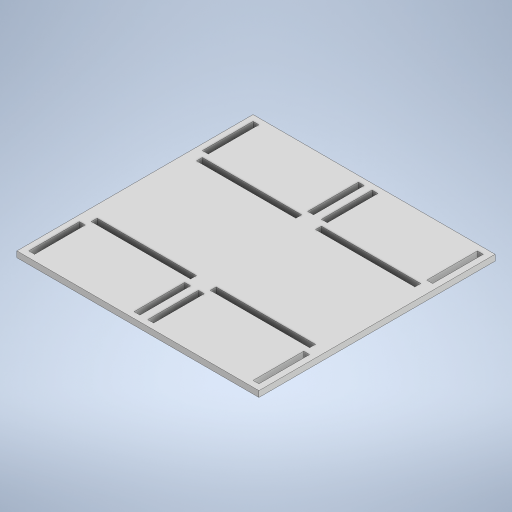
# Autodesk Inventor part: top
Saved by Autodesk Inventor 2023 (Build 270158000, 158)
## iProperties
Created: 2023-11-13
Part Number: top
Material: Generic
Document SubType Name: Modeling
Designer: Nate
Density: 1 g/cm^3
Appearance: Default
Mass: 45.5982 g
Surface Area: 339.233 cm^2
Volume: 45.5982 cm^3
Author: Nate
Autodesk Inventor part; units mm, degrees
ref_plane "YZ Plane" through (0, 0, 0) normal (1, 0, 0) x (0, 1, 0)
ref_plane "XZ Plane" through (0, 0, 0) normal (0, 1, 0) x (-1, 0, 0)
ref_plane "XY Plane" through (0, 0, 0) normal (0, 0, 1) x (1, 0, 0)
sketch "Sketch1" plane through (0, 0, 0) normal (0, 1, 0) x (-1, 0, 0)
  line L0 (0, 0) -> (127, 0)
  line L1 (127, 0) -> (127, -127)
  line L2 (127, -127) -> (0, -127)
  line L3 (0, -127) -> (0, 0)
  line L4 (123.825, 0) -> (127, 0)
  line L5 (127, 0) -> (127, -33.615)
  line L6 (127, -33.615) -> (123.825, -33.615)
  line L7 (123.825, -33.615) -> (123.825, 0)
  line L8 (123.825, -33.615) -> (70.363, -33.615)
  line L9 (70.363, -33.615) -> (70.363, -36.79)
  line L10 (70.363, -36.79) -> (127, -36.79)
  line L11 (70.363, -36.79) -> (67.188, -36.79)
  line L12 (67.188, -36.79) -> (67.188, 0)
  line L13 (67.188, 0) -> (70.363, 0)
  line L14 (70.363, 0) -> (70.363, -36.79)
  line L15 (127, -90.21) -> (67.188, -90.21)
  line L16 (67.188, -90.21) -> (67.188, -93.385)
  line L17 (67.188, -93.385) -> (127, -93.385)
  line L18 (127, -93.385) -> (127, -90.21)
  line L19 (127, -93.385) -> (123.825, -93.385)
  line L20 (123.825, -93.385) -> (123.825, -127)
  line L21 (123.825, -127) -> (127, -127)
  line L22 (127, -127) -> (127, -93.385)
  line L23 (25.4, 0) -> (6.35, 0)
  line L24 (25.4, -127) -> (6.35, -127)
  line L25 (67.188, -90.21) -> (70.363, -90.21)
  line L26 (70.363, -90.21) -> (70.363, -127)
  line L27 (70.363, -127) -> (67.188, -127)
  line L28 (67.188, -127) -> (67.188, -90.21)
  line L29 (67.188, -3.175) -> (70.363, -3.175)
  line L30 (70.363, -3.175) -> (70.363, -33.615)
  line L31 (70.363, -33.615) -> (67.188, -33.615)
  line L32 (67.188, -33.615) -> (67.188, -3.175)
  line L33 (73.538, -33.615) -> (123.825, -33.615)
  line L34 (123.825, -33.615) -> (123.825, -36.79)
  line L35 (123.825, -36.79) -> (73.538, -36.79)
  line L36 (127, -3.175) -> (123.825, -3.175)
  line L37 (123.825, -3.175) -> (123.825, -30.44)
  line L38 (123.825, -30.44) -> (127, -30.44)
  line L39 (127, -30.44) -> (127, -3.175)
  line L40 (123.825, -90.21) -> (81.7068, -90.21)
  line L41 (81.7068, -93.385) -> (123.825, -93.385)
  line L42 (123.825, -93.385) -> (123.825, -90.21)
  line L43 (123.825, -96.56) -> (127, -96.56)
  line L44 (127, -96.56) -> (127, -123.825)
  line L45 (127, -123.825) -> (123.825, -123.825)
  line L46 (123.825, -123.825) -> (123.825, -96.56)
  line L47 (70.363, -96.56) -> (67.188, -96.56)
  line L48 (67.188, -96.56) -> (67.188, -123.825)
  line L49 (67.188, -123.825) -> (70.363, -123.825)
  line L50 (70.363, -123.825) -> (70.363, -96.56)
  line L51 (70.363, -30.44) -> (67.188, -30.44)
  line L52 (22.225, 0) -> (9.525, 0)
  line L53 (9.525, -127) -> (22.225, -127)
  line L54 (127, 0) -> (130.175, 0)
  line L55 (130.175, 0) -> (130.175, -127)
  line L56 (130.175, -127) -> (127, -127)
  line L57 (127, -127) -> (127, 0)
  line L58 (3.175, 0) -> (0, 0)
  line L59 (0, 0) -> (0, -127)
  line L60 (0, -127) -> (3.175, -127)
  line L61 (3.175, -127) -> (3.175, 0)
  line L62 (62.987, 0) -> (62.987, -33.6042)
  line L63 (62.987, -33.6042) -> (59.812, -33.6042)
  line L64 (59.812, -33.6042) -> (59.812, -4.3263)
  line L65 (59.812, -33.6042) -> (6.35, -33.6042)
  line L66 (6.35, -33.6042) -> (6.35, -36.7792)
  line L67 (6.35, -36.7792) -> (62.987, -36.7792)
  line L68 (6.35, -36.7792) -> (3.175, -36.7792)
  line L69 (3.175, -36.7792) -> (3.175, -2.1822)
  line L70 (6.35, 0) -> (6.35, -36.7792)
  line L71 (3.175, -3.175) -> (6.35, -3.175)
  line L72 (6.35, -3.175) -> (6.35, -33.6042)
  line L73 (6.35, -33.6042) -> (3.175, -33.6042)
  line L74 (3.175, -33.6042) -> (3.175, -3.175)
  line L75 (59.812, -33.6042) -> (59.812, -36.7792)
  line L76 (62.987, -3.175) -> (59.812, -3.175)
  line L77 (59.812, -3.175) -> (59.812, -30.4292)
  line L78 (59.812, -30.4292) -> (62.987, -30.4292)
  line L79 (62.987, -30.4292) -> (62.987, -3.175)
  line L80 (6.35, -30.4292) -> (3.175, -30.4292)
  line L81 (62.987, -36.7792) -> (62.987, 0)
  line L82 (59.812, -3.175) -> (59.812, 0)
  line L83 (62.992, -127) -> (59.817, -127)
  line L84 (59.817, -127) -> (59.817, -90.2208)
  line L85 (59.817, -90.2208) -> (62.992, -90.2208)
  line L86 (62.992, -90.2208) -> (62.992, -127)
  line L87 (62.992, -93.3958) -> (3.175, -93.3958)
  line L88 (3.175, -93.3958) -> (3.175, -90.2208)
  line L89 (3.175, -90.2208) -> (62.992, -90.2208)
  line L90 (62.992, -90.2208) -> (62.992, -93.3958)
  line L91 (6.35, -90.2208) -> (3.175, -90.2208)
  line L92 (3.175, -90.2208) -> (3.175, -127)
  line L93 (3.175, -127) -> (6.35, -127)
  line L94 (6.35, -127) -> (6.35, -90.2208)
  line L95 (6.35, -123.825) -> (3.175, -123.825)
  line L96 (3.175, -123.825) -> (3.175, -96.5708)
  line L97 (3.175, -96.5708) -> (6.35, -96.5708)
  line L98 (6.35, -96.5708) -> (6.35, -123.825)
  line L99 (62.992, -123.825) -> (59.817, -123.825)
  line L100 (59.817, -123.825) -> (59.817, -96.5708)
  line L101 (59.817, -96.5708) -> (62.992, -96.5708)
  line L102 (62.992, -96.5708) -> (62.992, -123.825)
  point P0 (97.094, -33.615)
  point P1 (123.825, -110.1925)
  point P2 (123.825, -16.8075)
  point P3 (125.4125, 0)
  point P4 (125.4125, -3.175)
  point P5 (125.4125, -33.615)
  point P6 (70.363, -35.2025)
  point P7 (68.7755, -36.79)
  point P8 (68.7755, -33.615)
  point P9 (68.7755, 0)
  point P10 (68.7755, -3.175)
  point P11 (68.7755, -127)
  point P12 (68.7755, -123.825)
  point P13 (70.363, -93.385)
  point P14 (70.363, -30.44)
  point P15 (127, -96.56)
  point P16 (127, -30.44)
  point P17 (123.825, -33.615)
  point P18 (67.188, -96.56)
  point P19 (127, -93.385)
  point P20 (33.081, -33.6042)
  point P21 (59.812, -18.9652)
  point P22 (61.3995, -3.175)
  point P23 (61.3995, -33.6042)
  point P24 (6.35, -35.1917)
  point P25 (4.7625, -36.7792)
  point P26 (4.7625, -33.6042)
  point P27 (4.7625, -3.175)
  point P28 (59.817, -93.3958)
  point P29 (6.35, -93.3958)
  point P30 (3.175, -3.175)
  dimension "d0" = 127
  dimension "d2" = 127
  dimension "d5" = 33.615
  dimension "d6" = 33.615
  dimension "d7" = 53.462
  dimension "d8" = 53.462
  dimension "d9" = 3.175
  dimension "d10" = 3.175
  dimension "d11" = 3.175
  dimension "d12" = 3.175
  dimension "d13" = 3.175
  dimension "d14" = 3.175
  dimension "d28" = 3.175
  dimension "d29" = 3.175
  dimension "d30" = 3.175
  dimension "d32" = 3.175
  dimension "d33" = 3.175
  dimension "d34" = 3.175
  dimension "d35" = 3.175
  dimension "d36" = 3.175
  dimension "d37" = 3.175
  dimension "d38" = 3.175
  dimension "d57" = 3.175
  dimension "d58" = 3.175
  dimension "d90" = 53.462
  dimension "d91" = 3.175
  dimension "d92" = 3.175
  dimension "d93" = 3.175
  dimension "d94" = 3.175
  dimension "d96" = 3.175
  dimension "d97" = 3.175
  dimension "d98" = 0
  dimension "d99" = 3.175
  dimension "d100" = 3.175
  dimension "d101" = 33.6042
  dimension "d102" = 33.6042
  dimension "d103" = 53.467
  dimension "d104" = 0
  dimension "d105" = 0
  dimension "d106" = 0
  dimension "d107" = 3.175
  dimension "d108" = 3.175
  dimension "d109" = 3.175
  dimension "d110" = 3.175
  dimension "d111" = 3.175
  dimension "d112" = 3.175
  dimension "d113" = 3.175
  constraints: 206 end point, 44 parallel, 44 point on line, 27 horizontal, 26 perpendicular, 21 midpoint, 2 vertical
  measures "d0" distance between parallel lines of L2 L0
  measures "d2" distance between parallel lines of L1 L3
  measures "d5" distance from line of point (97.094, -33.615) L0
  measures "d6" distance between parallel lines of L2 L17
  measures "d7" distance from line of point (123.825, -110.192) L26
  measures "d8" distance from line of L14 point (123.825, -16.808)
  measures "d9" distance between parallel lines of L5 L7
  measures "d10" distance between parallel lines of L1 L20
  measures "d11" distance between parallel lines of L26 L28
  measures "d12" distance between parallel lines of L14 L12
  measures "d13" distance between parallel lines of L10 L8
  measures "d14" distance between parallel lines of L17 L15
  measures "d28" distance of point (125.412, 0) point (125.413, -3.175)
  measures "d29" vertical distance of point (125.413, -33.615) L38.end
  measures "d30" distance between parallel lines of L1 L34
  measures "d32" distance of point (68.775, -36.79) point (68.775, -33.615)
  measures "d33" distance of point (68.775, 0) point (68.775, -3.175)
  measures "d34" distance between parallel lines of L31 L51
  measures "d35" distance between parallel lines of L17 L47
  measures "d36" distance of point (68.775, -127) point (68.775, -123.825)
  measures "d37" distance between parallel lines of L1 L42
  measures "d38" distance between parallel lines of L43 L19
  measures "d57" distance between parallel lines of L55 L57
  measures "d58" distance between parallel lines of L61 L59
  measures "d90" distance from line of L70 point (59.812, -18.965)
  measures "d91" distance between parallel lines of L62 L64
  measures "d92" distance between parallel lines of L70 L69
  measures "d93" distance between parallel lines of L67 L65
  measures "d94" vertical distance of point (61.4, -33.604) L78.end
  measures "d96" distance of point (4.762, -36.779) point (4.762, -33.604)
  measures "d97" distance between parallel lines of L73 L80
  measures "d98" distance between parallel lines of L61 L69
  measures "d99" distance between parallel lines of L0 L71
  measures "d100" distance between parallel lines of L0 L76
  measures "d101" distance between parallel lines of L65 L0
  measures "d102" distance between parallel lines of L2 L87
  measures "d103" distance between parallel lines of L94 L84
  measures "d104" distance between parallel lines of L61 L92
  measures "d105" distance between parallel lines of L2 L93
  measures "d106" distance between parallel lines of L2 L83
  measures "d107" distance between parallel lines of L2 L99
  measures "d108" distance between parallel lines of L87 L101
  measures "d109" distance between parallel lines of L87 L97
  measures "d110" distance between parallel lines of L2 L95
  measures "d111" distance between parallel lines of L100 L102
  measures "d112" distance between parallel lines of L96 L98
  measures "d113" distance between parallel lines of L87 L89
extrude "Extrusion1" add sketch "Sketch1" along normal blind 3.175 contours L0 L61 L2 L3 | L0 L70 L71 L61 | L0 L82 L77 L64 L65 L70 | L61 L95 L94 L2 | L94 L87 L84 L2 | L70 L73 L61 L80 | L61 L87 L94 L97 | L66 L68 L61 L73 | L61 L89 L94 L87 | L0 L62 L76 L82 | L64 L78 L62 L63 | L63 L81 L67 L75 | L67 L81 L62 L0 L12 L11 L10 L1 L15 L16 L28 L2 L86 L85 L89 L61 L68 | L84 L99 L86 L2 | L87 L86 L101 L84 | L84 L85 L86 L87 | L0 L14 L29 L12 | L0 L7 L8 L14 | L28 L49 L26 L2 | L0 L1 L36 L7 | L51 L14 L31 L12 | L26 L17 L20 L2 | L54 L55 L56 L1 | L31 L9 L11 L12 | L20 L45 L1 L2 | L28 L17 L26 L47 | L38 L1 L6 L7 | L16 L15 L26 L17 | L6 L1 L10 L34 | L20 L17 L1 L43 | L42 L15 L1 L17
equation "\"d3\" = d41"
equation "\"d41\" = 3.175"
body "Solid1"
